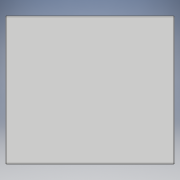
# Autodesk Inventor part: CD殼
Saved by Autodesk Inventor 2019 (Build 230136000, 136)
## iProperties
Created: 2019-01-19
Part Number: CD殼
Material: 一般
Document SubType Name: Modeling
Designer: j13tw
Density: 1 g/cm^3
Appearance: 預設
Author: j13tw
Autodesk Inventor part; units mm, degrees
ref_plane "YZ Plane" through (0, 0, 0) normal (1, 0, 0) x (0, 1, 0)
ref_plane "XZ Plane" through (0, 0, 0) normal (0, 1, 0) x (-1, 0, 0)
ref_plane "XY Plane" through (0, 0, 0) normal (0, 0, 1) x (1, 0, 0)
sketch "草圖1" plane through (0, 0, 0) normal (0, 0, 1) x (1, 0, 0)
  line L0 (0, 0) -> (142, 0)
  line L1 (142, 0) -> (142, 125)
  line L2 (142, 125) -> (0, 125)
  line L3 (0, 125) -> (0, 0)
  dimension "d0" = 125
  dimension "d1" = 142
  constraints: 8 end point, 2 parallel, 1 horizontal, 1 perpendicular
  measures "d0" distance of L0.end L1.end
  measures "d1" distance of L1.end L2.end
extrude "擠出1" add sketch "草圖1" along normal blind 10
fillet "圓角1" radius 1 4 edges at (0, 62.5, 10) (142, 62.5, 10) (142, 62.5, 0) (0, 62.5, 0)
fillet "圓角2" radius 1 16 edges at (0.2929, 125, 0.2929) (0, 125, 5) (0.2929, 125, 9.7071) (71, 125, 10) (141.7071, 125, 9.7071) (142, 125, 5) (141.7071, 125, 0.2929) (71, 125, 0) (141.7071, 0, 9.7071) (142, 0, 5) (141.7071, 0, 0.2929) (71, 0, 0) (0.2929, 0, 0.2929) (0, 0, 5) (0.2929, 0, 9.7071) (71, 0, 10)
